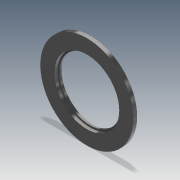
# Autodesk Inventor part: 4000120
Saved by Autodesk Inventor 2021 (Build 250183000, 183)
## iProperties
Created: 2003-05-27
Part Number: 4000120
Document SubType Name: Modeling
Designer: JLO
Material: 304L Stainless Steel
Description: QF50-200-BW
Density: 8.03 g/cm^3
Mass: 82.719 g
Surface Area: 66.2246 cm^2
Volume: 10.3012 cm^3
Appearance: Stainless - Brushed
Authority: QF50-200 SS BORED WELD FLANGE
Control State: 0
Master: False
Checked Out: False
Shininess: 64.0
Length Units: 11272
Angle Units: 11279
Time Units: 11290
Mass Units: 11286
Length Display Precision: 3
Angle Display Precision: 2
Compacted: True
Density: 0.0
Volumn: 0.0
Area: 0.0
PropertySet Name: Model Information
Author: JLO
Revision Number: D
Autodesk Inventor part; units mm, degrees
ref_plane "YZ Plane" through (0, 0, 0) normal (1, 0, 0) x (0, 1, 0)
ref_plane "XZ Plane" through (0, 0, 0) normal (0, 1, 0) x (-1, 0, 0)
ref_plane "XY Plane" through (0, 0, 0) normal (0, 0, 1) x (1, 0, 0)
sketch "Sketch2" plane through (0, 0, 0) normal (0, 0, 1) x (1, 0, 0)
  circle A0 centre (0, 0) radius 37.5031
  dimension "d0" = 75.0062
  constraints: 1 centre point, 1 coincident
  measures "d0" diameter of A0
extrude "Extrusion1" add sketch "Sketch2" against normal blind 3.048
sketch "Sketch3" plane through (0, 0, -3.048) normal (0, 0, -1) x (-1, 0, 0)
  circle A0 centre (0, 0) radius 37.5031 projected
extrude "Extrusion2" add sketch "Sketch3" along normal blind 2.032 draft -75
sketch "Sketch4" plane through (0, 0, 0) normal (0, 0, 1) x (1, 0, 0)
  circle A0 centre (0, 0) radius 37.5031 projected
  circle A1 centre (0, 0) radius 26.0985
  dimension "d5" = 52.197
  constraints: 1 centre point, 1 coincident, 1 concentric
  measures "d5" diameter of A1
extrude "Extrusion3" cut sketch "Sketch4" against normal blind 2.54 contours A1
sketch "Sketch5" plane through (0, 0, -5.08) normal (0, 0, -1) x (-1, 0, 0)
  circle A0 centre (0, 0) radius 29.9196 projected
  constraints: 1 coincident
hole "Hole1" at (0, 0, -5.08) direction (0, 0, 1) diameter 49.2252 end through all counterbore diameter 51.054 counterbore depth 1.27
body "Solid1"
